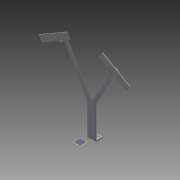
# Autodesk Inventor part: Feeder-Grabber_v2
Saved by Autodesk Inventor 2013 (Build 170138000, 138)
## iProperties
Created: 2013-01-21
Part Number: Feeder-Grabber_v2
Material: Generic
Document SubType Name: Sheet Metal
Designer: motoennies
Density: 1 g/cm^3
Sheet Metal Rule: Default
Author: motoennies
Autodesk Inventor part; units mm, degrees
ref_plane "YZ Plane" through (0, 0, 0) normal (1, 0, 0) x (0, 1, 0)
ref_plane "XZ Plane" through (0, 0, 0) normal (0, 1, 0) x (-1, 0, 0)
ref_plane "XY Plane" through (0, 0, 0) normal (0, 0, 1) x (1, 0, 0)
sketch "Sketch13" plane through (0, 0, 0) normal (0, 0, 1) x (1, 0, 0)
  line L0 (0, 0) -> (25.4, 0)
  line L1 (25.4, 0) -> (25.4, 101.6)
  line L2 (0, 0) -> (0, 101.6)
  line L3 (0, 101.6) -> (-76.2, 233.5823)
  line L4 (25.4, 101.6) -> (166.7245, 101.6) construction
  line L5 (25.4, 101.6) -> (101.6, 233.5823)
  line L6 (25.4, 101.6) -> (177.8, 101.6) construction
  line L7 (-76.2, 233.5823) -> (-65.2015, 239.9323)
  line L8 (101.6, 233.5823) -> (90.6015, 239.9323)
  line L9 (12.7, 105.003) -> (-65.2015, 239.9323)
  line L10 (12.7, 105.003) -> (-65.2015, 239.9323)
  line L11 (12.7, 105.003) -> (90.6015, 239.9323)
  circle A0 centre (12.7, 123.19) radius 139.7
  dimension "d54" = 25.4
  dimension "d55" = 101.6
  dimension "d56" = 150
  dimension "d59" = 152.4
  dimension "d63" = 152.4
  dimension "d64" = 60
  dimension "d65" = 12.7
  dimension "d66" = 12.7
  dimension "d82" = 279.4
  dimension "d83" = 123.19
  measures "d54" distance of L0.start L0.end
  measures "d55" distance of L0.end L1.end
  measures "d56" angle of L3 L2
  measures "d59" distance of L2.end L3.end
  measures "d63" distance of L1.end L5.end
  measures "d64" angle of L6 L5
  measures "d65" distance of L3.end L7.end
  measures "d66" distance from line of L2 L9.start
  measures "d82" diameter of A0
  measures "d83" distance from line of L0 A0.centre
extrude "Plate5" add sketch "Sketch13" along normal blind 3.048 contours L2 L3 A0 L9 L11 L5 L1 L0 | L3 L7 L9 A0 | A0 L11 L8 L5
sketch "Sketch14" plane through (89.0775, 237.2926, 0) normal (0.5, 0.8660254, 0) x (-0.8660254, 0.5, 0)
  line L0 (-12.7, 0) -> (0, 0)
  line L1 (0, 0) -> (0, 25.4)
  line L2 (0, 25.4) -> (-12.7, 25.4)
  line L3 (-12.7, 25.4) -> (-12.7, 0)
  constraints: 6 end point, 1 horizontal, 1 perpendicular, 1 vertical
edge flange "Flange4" height 25.4 angle 90 thickness 3.048 bend radius 3.048 thickness toward (0.5, 0.8660254, 0) relief straight relief width 3.048 relief depth 1.524 corner gap 3.048 corner form 0 edges at (96.1007, 236.7573, 3.048) (-70.7007, 236.7573, 3.048) wall of the first edge with corners at (100.076, 230.9426, 0) (89.0775, 237.2926, 0) (89.0775, 237.2926, 25.4) (100.076, 230.9426, 25.4)
bend "Bend4"
corner "Corner4"
sketch "Sketch15" plane through (100.076, 230.9426, 22.352) normal (0, 0, 1) x (1, 0, 0)
  line L0 (-10.9985, 6.35) -> (0, 0)
  line L1 (0, 0) -> (12.7, 21.997)
  line L2 (12.7, 21.997) -> (1.7015, 28.347)
  line L3 (1.7015, 28.347) -> (-10.9985, 6.35)
  constraints: 6 end point, 1 perpendicular, 2 other
edge flange "Flange5" height 25.4 angle 90 thickness 3.048 bend radius 3.048 thickness toward (0, 0, 1) relief straight relief width 3.048 relief depth 1.524 corner gap 3.048 corner form 0 edges at (96.1007, 236.7573, 25.4) (-70.7007, 236.7573, 25.4) wall of the first edge with corners at (89.0775, 237.2926, 22.352) (100.076, 230.9426, 22.352) (112.776, 252.9397, 22.352) (101.7775, 259.2897, 22.352)
bend "Bend5"
corner "Corner5"
sketch "Sketch16" plane through (-76.3775, 259.2897, 25.4) normal (0.8660254, 0.5, 0) x (0, 0, -1)
  line L0 (0, -19.304) -> (3.048, -19.304) projected
  line L1 (3.048, 0) -> (3.048, -19.304) projected
  line L2 (3.048, 0) -> (0, 0) projected
  line L3 (0, 0) -> (0, -19.304) projected
  point P0 (25.4, -262.7402)
extrude "Extrusion6" add sketch "Sketch16" along normal blind 38.1
sketch "Sketch17" plane through (101.7775, 259.2897, 22.352) normal (-0.8660254, 0.5, 0) x (0, 0, 1)
  line L0 (0, -19.304) -> (3.048, -19.304) projected
  line L1 (3.048, -19.304) -> (3.048, 0) projected
  line L2 (0, 0) -> (3.048, 0) projected
  line L3 (0, 0) -> (0, -19.304) projected
  point P0 (-22.352, -275.4402)
extrude "Extrusion7" add sketch "Sketch17" along normal blind 38.1
ref_plane "Work Plane1" through (0, 0, 25.4) normal (0, -1, 0) x (1, 0, 0)
sketch "Sketch20" plane through (0, 3.048, 3.048) normal (0, -1, 0) x (1, 0, 0)
  line L0 (25.4, 0) -> (0, 0)
  line L1 (0, 0) -> (0, -25.4)
  line L2 (0, -25.4) -> (25.4, -25.4)
  line L3 (25.4, -25.4) -> (25.4, 0)
  constraints: 6 end point, 1 horizontal, 1 perpendicular, 1 vertical
edge flange "Flange7" height 25.4 angle 90 thickness 3.048 bend radius 3.048 thickness toward (0, -1, 0) relief straight relief width 3.048 relief depth 1.524 edges at (12.7, 0, 0) wall of the first edge with corners at (25.4, 3.048, 3.048) (0, 3.048, 3.048) (0, 3.048, -22.352) (25.4, 3.048, -22.352)
bend "Bend7"
corner "Corner7"
sketch "Sketch21" plane through (0, 0, -22.352) normal (0, -1, 0) x (1, 0, 0)
  line L0 (25.4, 0) -> (0, 0) projected
  line L1 (25.4, 19.304) -> (25.4, 0) projected
  circle A0 centre (12.7, 9.652) radius 2.54
  point P0 (0, 22.352)
  dimension "d123" = 5.08
  dimension "d124" = 12.7
  dimension "d125" = 9.652
  constraints: 1 centre point
  measures "d123" diameter of A0
  measures "d124" distance from line of L1 A0.centre
  measures "d125" distance from line of L0 A0.centre
extrude "Cut3" cut sketch "Sketch21" against normal blind 3.048
sketch "Sketch22" plane through (-87.376, 252.9397, 22.352) normal (-0.8660254, -0.5, 0) x (0, 0, 1)
  line L0 (0, -19.304) -> (3.048, -19.304) projected
  line L1 (3.048, -19.304) -> (3.048, 0) projected
  line L2 (0, 0) -> (3.048, 0) projected
  line L3 (0, 0) -> (0, -19.304) projected
  point P0 (-22.352, -262.7402)
extrude "Extrusion8" add sketch "Sketch22" along normal blind 50.8
sketch "Sketch23" plane through (112.776, 252.9397, 25.4) normal (0.8660254, -0.5, 0) x (0, 0, -1)
  line L0 (0, -19.304) -> (3.048, -19.304) projected
  line L1 (3.048, 0) -> (3.048, -19.304) projected
  line L2 (3.048, 0) -> (0, 0) projected
  line L3 (0, 0) -> (0, -19.304) projected
  point P0 (25.4, -275.4402)
extrude "Extrusion9" add sketch "Sketch23" along normal blind 50.8
equation "\"d126\" = Thickness"
equation "\"d70\" = BendReliefWidth"
equation "\"d71\" = BendReliefDepth"
equation "\"d72\" = MinimumRemnant"
equation "\"d73\" = BendRadius"
equation "\"d76\" = BendRadius"
equation "\"d77\" = CornerReliefSize"
equation "\"d78\" = GapSize"
equation "\"d79\" = JacobiRadiusSize"
equation "\"d84\" = BendReliefWidth"
equation "\"d85\" = BendReliefDepth"
equation "\"d86\" = MinimumRemnant"
equation "\"d87\" = BendRadius"
equation "\"d90\" = BendRadius"
equation "\"d91\" = CornerReliefSize"
equation "\"d92\" = GapSize"
equation "\"d93\" = JacobiRadiusSize"
equation "\"d113\" = BendReliefWidth"
equation "\"d114\" = BendReliefDepth"
equation "\"d115\" = MinimumRemnant"
equation "\"d116\" = BendRadius"
equation "\"d119\" = BendRadius"
equation "\"d120\" = CornerReliefSize"
equation "\"d121\" = GapSize"
equation "\"d122\" = JacobiRadiusSize"
equation "\"BendRadius\" = Thickness"
equation "\"BendReliefWidth\" = Thickness"
equation "\"BendReliefDepth\" = 0.5 * Thickness"
equation "\"CornerReliefSize\" = 4 * Thickness"
equation "\"MinimumRemnant\" = 2 * Thickness"
equation "\"TransitionRadius\" = BendRadius"
equation "\"JacobiRadiusSize\" = BendRadius"
equation "\"GapSize\" = Thickness"
equation "\"d2\" = BendRadius"
equation "\"d69\" = BendRadius"
equation "\"Thickness\" = 3.048"
body "Solid3"
